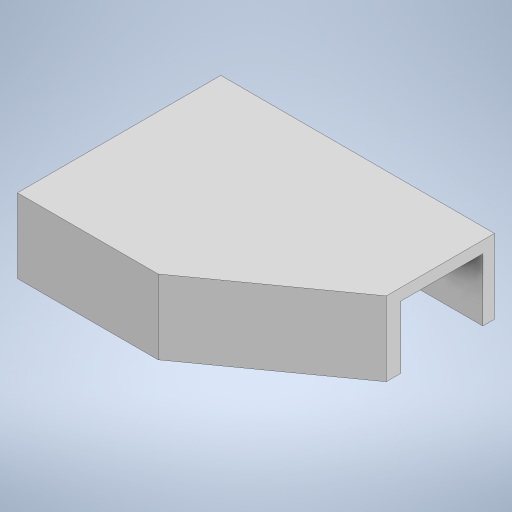
# Autodesk Inventor part: Cooling Fan Shroud
Saved by Autodesk Inventor 2023 (Build 270158000, 158)
## iProperties
Created: 2023-01-15
Part Number: Cooling Fan Shroud
Material: Generic
Document SubType Name: Modeling
Designer: Owner
Density: 1 g/cm^3
Appearance: Default
Author: Owner
Autodesk Inventor part; units mm, degrees
ref_plane "YZ Plane" through (0, 0, 0) normal (1, 0, 0) x (0, 1, 0)
ref_plane "XZ Plane" through (0, 0, 0) normal (0, 1, 0) x (-1, 0, 0)
ref_plane "XY Plane" through (0, 0, 0) normal (0, 0, 1) x (1, 0, 0)
sketch "Sketch1" plane through (0, 0, 0) normal (0, 1, 0) x (-1, 0, 0)
  line L0 (33.9701, -0.003) -> (69.9315, -0.003)
  line L1 (69.9315, -0.003) -> (69.9315, -52.003)
  line L2 (69.9315, -52.003) -> (-0.0685, -52.003)
  line L3 (-0.0685, -49.003) -> (69.9315, -49.003)
  line L4 (34.9315, -3.003) -> (69.9315, -3.003)
  line L5 (-0.0685, -28.003) -> (34.9315, -3.003)
  line L6 (29.7701, -3.003) -> (-0.0685, -24.3163)
  line L7 (-0.0685, -52.003) -> (-0.0685, -24.3163)
  line L8 (29.7701, -3.003) -> (33.9701, -0.003)
  point P0 (0, 0)
  dimension "d0" = 70
  dimension "d1" = 52
  dimension "d2" = 3
  dimension "d3" = 3
  dimension "d4" = 3
  dimension "d5" = 21
  constraints: 18 end point, 5 point on line, 4 parallel, 2 perpendicular, 1 horizontal
  measures "d0" distance of L1.end L2.end
  measures "d1" distance of L0.end L1.end
  measures "d2" distance between parallel lines of L2 L3
  measures "d3" distance between parallel lines of L4 L0
  measures "d4" distance between parallel lines of L6 L5
  measures "d5" distance of L3.start L5.start
extrude "Extrusion1" add sketch "Sketch1" against normal blind 19 contours L0 L1 L4 L5 L7 L6 L8 | L1 L2 L7 L3
extrude "Extrusion2" add sketch "Sketch1" against normal blind 3 contours L1 L3 L7 L5 L4
body "Solid1"
